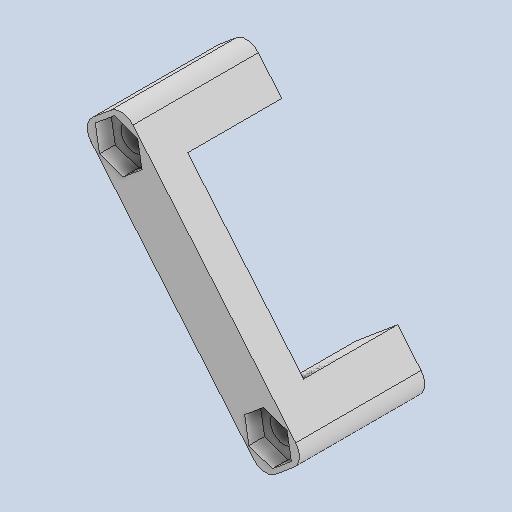
# Autodesk Inventor part: servo_holder
Saved by Autodesk Inventor 2024 (Build 280153000, 153)
## iProperties
Created: 2026-02-15
Part Number: servo_holder
Material: Generic
Document SubType Name: Modeling
Designer: SEMEN
Density: 1 g/cm^3
Appearance: Default
Author: SEMEN
Autodesk Inventor part; units mm, degrees
ref_plane "YZ Plane" through (0, 0, 0) normal (1, 0, 0) x (0, 1, 0)
sketch "Sketch1" plane through (0, 0, 0) normal (0, 0, 1) x (1, 0, 0)
  line L0 (91.0829, 58.2221) -> (71.5983, 81.4264) projected
  line L1 (73.9454, 78.6312) -> (81.7568, 85.1904) projected
  line L2 (96.5471, 67.5766) -> (88.7358, 61.0174) projected
  line L3 (71.5983, 81.4264) -> (69.6691, 83.7239)
  line L4 (69.6691, 83.7239) -> (75.0298, 88.2253)
  line L5 (75.0298, 88.2253) -> (79.3061, 83.1326)
  line L6 (91.0829, 58.2221) -> (93.0121, 55.9247)
  line L7 (93.0121, 55.9247) -> (98.3728, 60.4261)
  line L8 (98.3728, 60.4261) -> (94.0965, 65.5188)
  line L9 (81.3406, 69.8243) -> (102.4069, 87.5137) construction
  line L10 (91.726, 57.4563) -> (90.0029, 56.0094) projected
  line L11 (95.6925, 58.1754) -> (91.4161, 63.2681) construction
  line L12 (72.3494, 85.9746) -> (76.6258, 80.8819) construction
  point P0 (0, 0)
  point P1 (93.5543, 60.7217)
  point P2 (74.4876, 83.4282)
  dimension "d0" = 2
  dimension "d1" = 7
  constraints: 18 end point, 7 point on line, 5 midpoint, 5 perpendicular, 1 other
  measures "d0" distance between parallel lines of L7 L10
  measures "d1" distance between parallel lines of L8 L0
ref_plane "Work Plane1" through (72.2806, 68.9104, 57.5461) normal (0, 0, 1) x (0.7658175, 0.643058, 0)
ref_plane "Work Plane2" through (75.6298, 74.8001, 12) normal (0, 0, 1) x (0.7658175, 0.643058, 0)
extrude "Extrusion1" add sketch "Sketch1" along normal up to surface (12 mm away)
sketch "Sketch2" plane through (98.3728, 60.4261, 12) normal (0, 0, 1) x (0.7658175, 0.643058, 0)
  line L0 (0, 0) -> (0, 6.65) projected
  line L1 (-7, 29.65) -> (-7, 36.3) projected
  line L2 (0, 0) -> (-7, 0)
  line L3 (-7, 0) -> (-7, 36.3)
  line L4 (-7, 36.3) -> (0, 36.3)
  line L5 (0, 36.3) -> (0, 0)
  point P0 (-114.1931, 16.9841)
  point P1 (0, 6.65)
  point P2 (-7, 29.65)
  constraints: 8 end point, 2 parallel, 1 horizontal, 1 perpendicular
extrude "Extrusion2" add sketch "Sketch2" along normal blind 4
hole "Hole1" at (74.4876, 83.4282, 0) at (93.5543, 60.7217, 0) direction (0, 0, 1) diameter 3.4 end through all clearance for "Countersunk Head GOST 12876-67" size "M3" standard "GOST"
fillet "Fillet1" radius 2 8 edges at (93.0121, 55.9247, 14) (93.0121, 55.9247, 6) (98.3728, 60.4261, 14) (98.3728, 60.4261, 6) (75.0298, 88.2253, 14) (75.0298, 88.2253, 6) (69.6691, 83.7239, 14) (69.6691, 83.7239, 6)
sketch "Sketch3" plane through (98.3728, 60.4261, 16) normal (0, 0, 1) x (0.7658175, 0.643058, 0)
  circle A0 centre (-3.5, 3.325) radius 1.7 projected
  circle A1 centre (-3.5, 32.975) radius 1.7 projected
  line L0 (-1.9123, 6.075) -> (-0.3246, 3.325)
  line L1 (-0.3246, 3.325) -> (-1.9123, 0.575)
  line L2 (-1.9123, 0.575) -> (-5.0877, 0.575)
  line L3 (-5.0877, 0.575) -> (-6.6754, 3.325)
  line L4 (-6.6754, 3.325) -> (-5.0877, 6.075)
  line L5 (-5.0877, 6.075) -> (-1.9123, 6.075)
  line L6 (-1.9123, 30.225) -> (-5.0877, 30.225)
  line L7 (-5.0877, 30.225) -> (-6.6754, 32.975)
  line L8 (-6.6754, 32.975) -> (-5.0877, 35.725)
  line L9 (-5.0877, 35.725) -> (-1.9123, 35.725)
  line L10 (-1.9123, 35.725) -> (-0.3246, 32.975)
  line L11 (-0.3246, 32.975) -> (-1.9123, 30.225)
  line L12 (-5, 0) -> (-2, 0) projected
  point P0 (-114.1931, 16.9841)
  point P1 (-3.5, 3.325)
  point P2 (-3.5, 32.975)
  dimension "d14" = 5.5
  dimension "d15" = 5.5
  constraints: 24 end point, 2 coincident, 2 parallel, 26 other
  measures "d14" distance between parallel lines of L2 L5
  measures "d15" distance between parallel lines of L9 L6
extrude "Extrusion3" cut sketch "Sketch3" against normal blind 2
body "Solid1"
